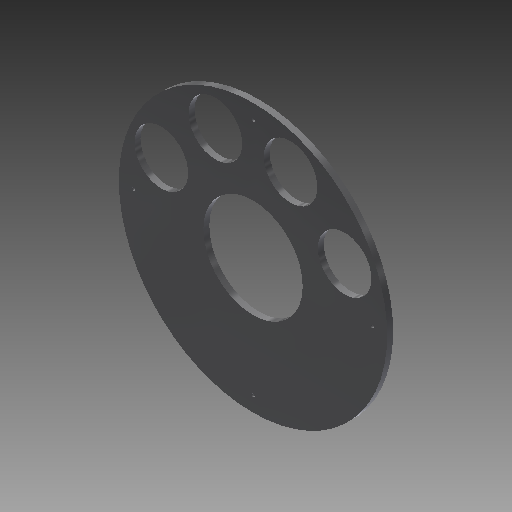
# Autodesk Inventor part: Диск_фиксирующий
Saved by Autodesk Inventor 2022 (Build 260153000, 153)
## iProperties
RuleStatus: InUse
Part Number: Диск_фиксирующий
Checked By: Якушев
Engr Approved By: Малов
Material: По умолчанию1
Document SubType Name: Modeling
Mfg Approved By: Судаков
Designer: Смирнов
Density: 1 g/cm^3
Appearance: Гладкий — нейтральный серый
AfterMaterialChange0: Материал
BeforeDocSave0: Материал
AfterAnyiPropertyChange0: Материал
Материал: По умолчанию1
Author: Смирнов
Autodesk Inventor part; units mm, degrees
ref_plane "YZ Plane" through (0, 0, 0) normal (1, 0, 0) x (0, 1, 0)
ref_plane "XZ Plane" through (0, 0, 0) normal (0, 1, 0) x (-1, 0, 0)
ref_plane "XY Plane" through (0, 0, 0) normal (0, 0, 1) x (1, 0, 0)
ref_plane "РабПлоскость1" through (0, 120, 53) normal (0, 0, 1) x (-1, 0, 0)
sketch "Эскиз1" plane through (0, 120, 53) normal (0, 0, 1) x (-1, 0, 0)
  circle A0 centre (0, 120) radius 135 projected
  circle A1 centre (0, 0) radius 1.6 projected
  circle A2 centre (-120, 120) radius 1.6 projected
  circle A3 centre (120, 120) radius 1.6 projected
  circle A4 centre (0, 240) radius 1.6 projected
  circle A5 centre (0, 120) radius 135 projected
  circle A6 centre (37.8353, 26.3544) radius 27 projected
  circle A7 centre (92.2681, 78.9196) radius 27 projected
  circle A8 centre (-37.8353, 26.3544) radius 27 projected
  circle A9 centre (-92.2681, 78.9196) radius 27 projected
  circle A10 centre (0, 120) radius 50 projected
  circle A11 centre (48.4361, 96.1266) radius 1.7 projected
  circle A12 centre (3.5431, 66.1164) radius 1.7 projected
  circle A13 centre (-44.8931, 89.9898) radius 1.7 projected
  circle A14 centre (-48.4361, 143.8734) radius 1.7 projected
  circle A15 centre (-3.5431, 173.8836) radius 1.7 projected
  circle A16 centre (44.8931, 150.0102) radius 1.7 projected
extrude "Выдавливание1" add sketch "Эскиз1" along normal blind 6 contours A0 | A10 | A11 | A12 | A13 | A14 | A15 | A16
sketch "Эскиз2" plane through (0, 0, 59) normal (0, 0, 1) x (1, 0, 0)
  circle A0 centre (0, 0) radius 50 projected
extrude "Выдавливание2" cut sketch "Эскиз2" against normal through all
